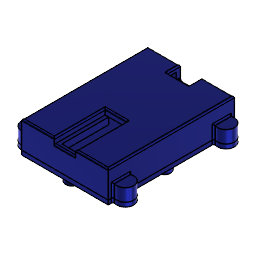
breadboard_case_CAD_v1 (Autodesk Fusion 360 design; units mm, degrees)
Autodesk Fusion 360 part; units mm, degrees
note: some values were not read from the file. Set by a fixed rule: which face or edge a step refers to.
(part 1 of 2)
sketch "breadboard_base" plane through (0, 0, 0) normal (0, 0, 1) x (1, 0, 0)
  line L0 (-27.2, 41.115) -> (27.2, 41.115)
  line L1 (27.2, 41.115) -> (27.2, -41.115)
  line L2 (27.2, -41.115) -> (-27.2, -41.115)
  line L3 (-27.2, -41.115) -> (-27.2, 41.115)
  dimension "d1" = 54.4
  dimension "d2" = 82.23
  dimension "d5" = 41.115
  dimension "d7" = 27.2
  constraint horizontal L0
  constraint vertical L1
  constraint horizontal L2
  constraint vertical L3
  measures "d1" distance of L0.start L0.end
  measures "d2" distance of L0.start L2.end
  measures "d5" distance of origin L0
  measures "d7" distance of origin L3
extrude "Extrude1" add sketch "breadboard_base" along normal blind 10 makes body 1
sketch "ravine_base" plane through (0, 0, 10) normal (0, 0, 1) x (-1, 0, 0)
  line L0 (27.2, 41.115) -> (-27.2, 41.115)
  line L1 (-27.2, 41.115) -> (-27.2, -41.115)
  line L2 (-27.2, -41.115) -> (27.2, -41.115)
  line L3 (27.2, -41.115) -> (27.2, 41.115)
  line L4 (1.5, -41.115) -> (-1.5, -41.115)
  line L5 (-1.5, -41.115) -> (-1.5, 41.115)
  line L6 (-1.5, 41.115) -> (1.5, 41.115)
  line L7 (1.5, 41.115) -> (1.5, -41.115)
  line L8 (0, -1.75) -> (0, -22.5)
  dimension "ravine_width" = 3
  constraint horizontal L4
  constraint vertical L5
  constraint horizontal L6
  constraint vertical L7
  constraint coincident L0 L5.end
  constraint coincident L2 L4.start
  constraint symmetric L5 L7 L8
  measures "ravine_width" distance of L5 L7
extrude "Extrude2" cut sketch "ravine_base" against normal blind 3 contours L0 L2 L4 L5 L6 L7 bodies 1
sketch "tab_base" plane through (0, 0, 0) normal (0, 0, 1) x (1, 0, 0)
  line L0 (-27.2, 41.115) -> (27.2, 41.115)
  line L1 (-27.2, -41.115) -> (-27.2, 41.115)
  line L2 (27.2, 41.115) -> (27.2, -41.115)
  line L3 (27.2, -41.115) -> (-27.2, -41.115)
  line L4 (1.5, 41.115) -> (1.5, -41.115)
  line L5 (1.5, -41.115) -> (27.2, -41.115)
  line L6 (1.5, -41.115) -> (-1.5, -41.115)
  line L7 (1.5, -41.115) -> (-1.5, -41.115)
  line L8 (-1.5, -41.115) -> (-1.5, -42.615)
  line L9 (-1.5, -42.615) -> (1.5, -42.615)
  line L10 (1.5, -42.615) -> (1.5, -41.115)
  line L11 (24.2, -41.115) -> (21.2, -41.115)
  line L12 (21.2, -41.115) -> (21.2, -42.615)
  line L13 (21.2, -42.615) -> (24.2, -42.615)
  line L14 (24.2, -42.615) -> (24.2, -41.115)
  line L15 (-21.2, -41.115) -> (-24.2, -41.115)
  line L16 (-24.2, -41.115) -> (-24.2, -42.615)
  line L17 (-24.2, -42.615) -> (-21.2, -42.615)
  line L18 (-21.2, -42.615) -> (-21.2, -41.115)
  line L19 (-27.2, -28.115) -> (-28.7, -28.115)
  line L20 (-28.7, -28.115) -> (-28.7, -25.115)
  line L21 (-28.7, -25.115) -> (-27.2, -25.115)
  line L22 (-27.2, -25.115) -> (-27.2, -28.115)
  line L23 (-27.2, 25.615) -> (-28.7, 25.615)
  line L24 (-28.7, 25.615) -> (-28.7, 28.615)
  line L25 (-28.7, 28.615) -> (-27.2, 28.615)
  line L26 (-27.2, 28.615) -> (-27.2, 25.615)
  dimension "d82" = 1.5
  dimension "d83" = 3
  dimension "d84" = 1.5
  dimension "d85" = 3
  dimension "d86" = 3
  dimension "d87" = 3
  dimension "d88" = 1.5
  dimension "d89" = 13
  dimension "d90" = 3
  dimension "d91" = 1.5
  dimension "d92" = 12.5
  dimension "d93" = 1.5
  dimension "d94" = 3
  constraint horizontal L7
  constraint vertical L8
  constraint horizontal L9
  constraint vertical L10
  constraint coincident L4.end L5.start
  constraint horizontal L11
  constraint vertical L12
  constraint horizontal L13
  constraint vertical L14
  constraint coincident L3 L11.start
  constraint horizontal L15
  constraint vertical L16
  constraint horizontal L17
  constraint vertical L18
  constraint coincident L3 L15.start
  constraint horizontal L19
  constraint vertical L20
  constraint horizontal L21
  constraint vertical L22
  constraint coincident L1 L19.start
  constraint horizontal L23
  constraint vertical L24
  constraint horizontal L25
  constraint vertical L26
  constraint coincident L1 L23.start
  measures "d82" distance of L6.end L8.end
  measures "d83" distance of L2.end L11.start
  measures "d84" distance of L11.end L12.end
  measures "d85" distance of L12.end L13.end
  measures "d86" distance of L1.start L15.end
  measures "d87" distance of L16.end L17.end
  measures "d88" distance of L15.start L17.end
  measures "d89" distance of L1.start L19
  measures "d90" distance of L19.end L20.end
  measures "d91" distance of L19.start L19.end
  measures "d92" distance of L0.start L25.end
  measures "d93" distance of L24.end L25.end
  measures "d94" distance of L23.end L24.end
extrude "Extrude3" add sketch "tab_base" along normal blind 5.1 contours L1 L23 L24 L25 L26 | L3 L6 L7 L8 L9 L10 | L3 L5 L11 L12 L13 L14 | L1 L19 L20 L21 L22 | L3 L15 L16 L17 L18 bodies 1
sketch "all_points" plane through (0, 0, 10) normal (0, 0, 1) x (-1, 0, 0)
  line L0 (1.5, 41.115) -> (1.5, -41.115)
  line L1 (1.5, -41.115) -> (27.2, -41.115)
  line L2 (27.2, -41.115) -> (27.2, 41.115)
  line L3 (27.2, 41.115) -> (1.5, 41.115)
  line L4 (0, 0) -> (27.2, 0) construction
  line L5 (-1.75, 0) -> (-22.5, 0)
  line L6 (0, -1.75) -> (0, -22.5)
  point P0 (3.8, -1.27)
  point P1 (6.34, -1.27)
  point P2 (8.88, -1.27)
  point P3 (11.42, -1.27)
  point P4 (13.96, -1.27)
  point P5 (3.8, -3.81)
  point P6 (6.34, -3.81)
  point P7 (8.88, -3.81)
  point P8 (11.42, -3.81)
  point P9 (13.96, -3.81)
  point P10 (3.8, -6.35)
  point P11 (6.34, -6.35)
  point P12 (8.88, -6.35)
  point P13 (11.42, -6.35)
  point P14 (13.96, -6.35)
  point P15 (3.8, -8.89)
  point P16 (6.34, -8.89)
  point P17 (8.88, -8.89)
  point P18 (11.42, -8.89)
  point P19 (13.96, -8.89)
  point P20 (3.8, -11.43)
  point P21 (6.34, -11.43)
  point P22 (8.88, -11.43)
  point P23 (11.42, -11.43)
  point P24 (13.96, -11.43)
  point P25 (3.8, -13.97)
  point P26 (6.34, -13.97)
  point P27 (8.88, -13.97)
  point P28 (11.42, -13.97)
  point P29 (13.96, -13.97)
  point P30 (3.8, -16.51)
  point P31 (6.34, -16.51)
  point P32 (8.88, -16.51)
  point P33 (11.42, -16.51)
  point P34 (13.96, -16.51)
  point P35 (3.8, -19.05)
  point P36 (6.34, -19.05)
  point P37 (8.88, -19.05)
  point P38 (11.42, -19.05)
  point P39 (13.96, -19.05)
  point P40 (3.8, -21.59)
  point P41 (6.34, -21.59)
  point P42 (8.88, -21.59)
  point P43 (11.42, -21.59)
  point P44 (13.96, -21.59)
  point P45 (3.8, -24.13)
  point P46 (6.34, -24.13)
  point P47 (8.88, -24.13)
  point P48 (11.42, -24.13)
  point P49 (13.96, -24.13)
  point P50 (3.8, -26.67)
  point P51 (6.34, -26.67)
  point P52 (8.88, -26.67)
  point P53 (11.42, -26.67)
  point P54 (13.96, -26.67)
  point P55 (3.8, -29.21)
  point P56 (6.34, -29.21)
  point P57 (8.88, -29.21)
  point P58 (11.42, -29.21)
  point P59 (13.96, -29.21)
  point P60 (3.8, -31.75)
  point P61 (6.34, -31.75)
  point P62 (8.88, -31.75)
  point P63 (11.42, -31.75)
  point P64 (13.96, -31.75)
  point P65 (3.8, -34.29)
  point P66 (6.34, -34.29)
  point P67 (8.88, -34.29)
  point P68 (11.42, -34.29)
  point P69 (13.96, -34.29)
  point P70 (3.8, -36.83)
  point P71 (6.34, -36.83)
  point P72 (8.88, -36.83)
  point P73 (11.42, -36.83)
  point P74 (13.96, -36.83)
  point P75 (20.71, 0)
  point P76 (20.71, -5.08)
  point P77 (23.25, -5.08)
  point P78 (20.71, -2.54)
  point P79 (23.25, -2.54)
  point P80 (23.25, 0)
  point P81 (20.71, 2.54)
  point P82 (23.25, 2.54)
  point P83 (20.71, 5.08)
  point P84 (23.25, 5.08)
  point P85 (23.25, -35.56)
  point P86 (23.25, -27.94)
  point P87 (20.71, -25.4)
  point P88 (23.25, -30.48)
  point P89 (20.71, -30.48)
  point P90 (23.25, -33.02)
  point P91 (20.71, -27.94)
  point P92 (20.71, -35.56)
  point P93 (23.25, -25.4)
  point P94 (20.71, -33.02)
  point P95 (23.25, -20.32)
  point P96 (23.25, -12.7)
  point P97 (20.71, -10.16)
  point P98 (23.25, -15.24)
  point P99 (20.71, -15.24)
  point P100 (23.25, -17.78)
  point P101 (20.71, -12.7)
  point P102 (20.71, -20.32)
  point P103 (23.25, -10.16)
  point P104 (20.71, -17.78)
  point P105 (23.25, 10.16)
  point P106 (23.25, 17.78)
  point P107 (20.71, 20.32)
  point P108 (23.25, 15.24)
  point P109 (20.71, 15.24)
  point P110 (23.25, 12.7)
  point P111 (20.71, 17.78)
  point P112 (20.71, 10.16)
  point P113 (23.25, 20.32)
  point P114 (20.71, 12.7)
  point P115 (23.25, 25.4)
  point P116 (23.25, 33.02)
  point P117 (20.71, 35.56)
  point P118 (23.25, 30.48)
  point P119 (20.71, 30.48)
  point P120 (23.25, 27.94)
  point P121 (20.71, 33.02)
  point P122 (20.71, 25.4)
  point P123 (23.25, 35.56)
  point P124 (20.71, 27.94)
  point P125 (6.34, 26.67)
  point P126 (13.96, 16.51)
  point P127 (3.8, 29.21)
  point P128 (13.96, 19.05)
  point P129 (6.34, 11.43)
  point P130 (8.88, 6.35)
  point P131 (3.8, 13.97)
  point P132 (6.34, 19.05)
  point P133 (3.8, 36.83)
  point P134 (8.88, 31.75)
  point P135 (13.96, 21.59)
  point P136 (3.8, 19.05)
  point P137 (6.34, 13.97)
  point P138 (3.8, 24.13)
  point P139 (13.96, 3.81)
  point P140 (6.34, 34.29)
  point P141 (13.96, 31.75)
  point P142 (6.34, 3.81)
  point P143 (13.96, 24.13)
  point P144 (11.42, 1.27)
  point P145 (13.96, 6.35)
  point P146 (8.88, 16.51)
  point P147 (11.42, 21.59)
  point P148 (6.34, 8.89)
  point P149 (6.34, 21.59)
  point P150 (6.34, 1.27)
  point P151 (8.88, 26.67)
  point P152 (11.42, 6.35)
  point P153 (13.96, 1.27)
  point P154 (3.8, 3.81)
  point P155 (3.8, 8.89)
  point P156 (8.88, 29.21)
  point P157 (6.34, 24.13)
  point P158 (13.96, 36.83)
  point P159 (11.42, 34.29)
  point P160 (8.88, 24.13)
  point P161 (3.8, 11.43)
  point P162 (11.42, 36.83)
  point P163 (11.42, 24.13)
  point P164 (11.42, 13.97)
  point P165 (13.96, 8.89)
  point P166 (6.34, 29.21)
  point P167 (6.34, 6.35)
  point P168 (8.88, 36.83)
  point P169 (11.42, 31.75)
  point P170 (3.8, 6.35)
  point P171 (8.88, 11.43)
  point P172 (6.34, 16.51)
  point P173 (3.8, 31.75)
  point P174 (13.96, 26.67)
  point P175 (8.88, 3.81)
  point P176 (8.88, 19.05)
  point P177 (8.88, 1.27)
  point P178 (13.96, 13.97)
  point P179 (8.88, 13.97)
  point P180 (6.34, 31.75)
  point P181 (8.88, 8.89)
  point P182 (11.42, 26.67)
  point P183 (3.8, 1.27)
  point P184 (11.42, 19.05)
  point P185 (13.96, 29.21)
  point P186 (11.42, 29.21)
  point P187 (3.8, 21.59)
  point P188 (13.96, 11.43)
  point P189 (11.42, 11.43)
  point P190 (13.96, 34.29)
  point P191 (3.8, 34.29)
  point P192 (11.42, 8.89)
  point P193 (11.42, 16.51)
  point P194 (11.42, 3.81)
  point P195 (3.8, 26.67)
  point P196 (8.88, 21.59)
  point P197 (8.88, 34.29)
  point P198 (6.34, 36.83)
  point P199 (3.8, 16.51)
  point P200 (-23.25, -15.24)
  point P201 (-3.8, 1.27)
  point P202 (-3.8, -29.21)
  point P203 (-23.25, -10.16)
  point P204 (-8.88, -24.13)
  point P205 (-8.88, 21.59)
  point P206 (-6.34, -13.97)
  point P207 (-20.71, 10.16)
  point P208 (-23.25, 15.24)
  point P209 (-6.34, 29.21)
  point P210 (-11.42, -24.13)
  point P211 (-23.25, -25.4)
  point P212 (-13.96, -11.43)
  point P213 (-3.8, -13.97)
  point P214 (-3.8, -8.89)
  point P215 (-3.8, -16.51)
  point P216 (-20.71, -35.56)
  point P217 (-13.96, -29.21)
  point P218 (-23.25, -30.48)
  point P219 (-3.8, -3.81)
  point P220 (-6.34, -19.05)
  point P221 (-20.71, -30.48)
  point P222 (-11.42, -36.83)
  point P223 (-6.34, -16.51)
  point P224 (-20.71, -27.94)
  point P225 (-6.34, 16.51)
  point P226 (-11.42, -31.75)
  point P227 (-20.71, 12.7)
  point P228 (-11.42, -6.35)
  point P229 (-13.96, -19.05)
  point P230 (-11.42, 31.75)
  point P231 (-20.71, 15.24)
  point P232 (-11.42, 8.89)
  point P233 (-13.96, -13.97)
  point P234 (-13.96, -16.51)
  point P235 (-8.88, -26.67)
  point P236 (-3.8, -34.29)
  point P237 (-3.8, 26.67)
  point P238 (-13.96, -26.67)
  point P239 (-13.96, 21.59)
  point P240 (-20.71, 17.78)
  point P241 (-3.8, 13.97)
  point P242 (-8.88, -31.75)
  point P243 (-6.34, -36.83)
  point P244 (-3.8, -19.05)
  point P245 (-20.71, -12.7)
  point P246 (-23.25, -35.56)
  point P247 (-11.42, -21.59)
  point P248 (-3.8, -26.67)
  point P249 (-13.96, -21.59)
  point P250 (-3.8, -6.35)
  point P251 (-20.71, -15.24)
  point P252 (-8.88, -21.59)
  point P253 (-6.34, -26.67)
  point P254 (-13.96, -36.83)
  point P255 (-11.42, -29.21)
  point P256 (-6.34, -34.29)
  point P257 (-3.8, 6.35)
  point P258 (-3.8, -1.27)
  point P259 (-20.71, -20.32)
  point P260 (-6.34, -21.59)
  point P261 (-8.88, -3.81)
  point P262 (-11.42, 29.21)
  point P263 (-13.96, -34.29)
  point P264 (-8.88, 8.89)
  point P265 (-23.25, 17.78)
  point P266 (-23.25, -12.7)
  point P267 (-3.8, -11.43)
  point P268 (-8.88, -16.51)
  point P269 (-3.8, 3.81)
  point P270 (-13.96, -31.75)
  point P271 (-11.42, -16.51)
  point P272 (-8.88, -19.05)
  point P273 (-8.88, -36.83)
  point P274 (-20.71, -25.4)
  point P275 (-23.25, -17.78)
  point P276 (-23.25, -27.94)
  point P277 (-6.34, -29.21)
  point P278 (-23.25, -33.02)
  point P279 (-23.25, -20.32)
  point P280 (-20.71, -33.02)
  point P281 (-23.25, 20.32)
  point P282 (-11.42, -11.43)
  point P283 (-6.34, 24.13)
  point P284 (-3.8, -21.59)
  point P285 (-3.8, 21.59)
  point P286 (-13.96, 34.29)
  point P287 (-6.34, 8.89)
  point P288 (-20.71, 20.32)
  point P289 (-11.42, -8.89)
  point P290 (-13.96, -24.13)
  point P291 (-8.88, -13.97)
  point P292 (-8.88, 29.21)
  point P293 (-6.34, -11.43)
  point P294 (-11.42, -13.97)
  point P295 (-23.25, 12.7)
  point P296 (-11.42, 19.05)
  point P297 (-11.42, 24.13)
  point P298 (-3.8, -36.83)
  point P299 (-20.71, 27.94)
  point P300 (-6.34, 21.59)
  point P301 (-20.71, 30.48)
  point P302 (-13.96, -1.27)
  point P303 (-11.42, 16.51)
  point P304 (-13.96, -6.35)
  point P305 (-13.96, 11.43)
  point P306 (-8.88, 16.51)
  point P307 (-11.42, 34.29)
  point P308 (-6.34, 36.83)
  point P309 (-23.25, 30.48)
  point P310 (-13.96, 24.13)
  point P311 (-6.34, 31.75)
  point P312 (-20.71, 35.56)
  point P313 (-3.8, -24.13)
  point P314 (-11.42, 3.81)
  point P315 (-6.34, 19.05)
  point P316 (-8.88, 11.43)
  point P317 (-3.8, 24.13)
  point P318 (-8.88, 34.29)
  point P319 (-23.25, -5.08)
  point P320 (-8.88, -34.29)
  point P321 (-8.88, 31.75)
  point P322 (-23.25, 33.02)
  point P323 (-6.34, -8.89)
  point P324 (-8.88, 19.05)
  point P325 (-8.88, 26.67)
  point P326 (-8.88, -29.21)
  point P327 (-6.34, 26.67)
  point P328 (-13.96, 26.67)
  point P329 (-6.34, -24.13)
  point P330 (-6.34, -31.75)
  point P331 (-11.42, -19.05)
  point P332 (-8.88, 36.83)
  point P333 (-11.42, 21.59)
  point P334 (-11.42, 6.35)
  point P335 (-20.71, 5.08)
  point P336 (-8.88, 24.13)
  point P337 (-11.42, -34.29)
  point P338 (-13.96, 8.89)
  point P339 (-3.8, 19.05)
  point P340 (-20.71, 0)
  point P341 (-3.8, 36.83)
  point P342 (-20.71, -17.78)
  point P343 (-13.96, 31.75)
  point P344 (-13.96, 13.97)
  point P345 (-23.25, 2.54)
  point P346 (-11.42, -26.67)
  point P347 (-20.71, -10.16)
  point P348 (-8.88, -11.43)
  point P349 (-3.8, 16.51)
  point P350 (-20.71, -5.08)
  point P351 (-23.25, 10.16)
  point P352 (-3.8, -31.75)
  point P353 (-13.96, 19.05)
  point P354 (-20.71, 25.4)
  point P355 (-20.71, 33.02)
  point P356 (-13.96, 36.83)
  point P357 (-11.42, 36.83)
  point P358 (-11.42, 26.67)
  point P359 (-6.34, 34.29)
  point P360 (-11.42, 11.43)
  point P361 (-6.34, 11.43)
  point P362 (-8.88, 13.97)
  point P363 (-3.8, 31.75)
  point P364 (-11.42, 13.97)
  point P365 (-23.25, 5.08)
  point P366 (-23.25, 27.94)
  point P367 (-13.96, 29.21)
  point P368 (-3.8, 8.89)
  point P369 (-3.8, 29.21)
  point P370 (-23.25, 25.4)
  point P371 (-3.8, 11.43)
  point P372 (-3.8, 34.29)
  point P373 (-6.34, 13.97)
  point P374 (-13.96, 6.35)
  point P375 (-8.88, 3.81)
  point P376 (-8.88, -6.35)
  point P377 (-13.96, 16.51)
  point P378 (-11.42, 1.27)
  point P379 (-23.25, 35.56)
  point P380 (-13.96, 1.27)
  point P381 (-8.88, 1.27)
  point P382 (-13.96, -3.81)
  point P383 (-6.34, -3.81)
  point P384 (-23.25, 0)
  point P385 (-8.88, -1.27)
  point P386 (-6.34, -6.35)
  point P387 (-23.25, -2.54)
  point P388 (-6.34, 3.81)
  point P389 (-6.34, 1.27)
  point P390 (-6.34, -1.27)
  point P391 (-20.71, 2.54)
  point P392 (-13.96, 3.81)
  point P393 (-13.96, -8.89)
  point P394 (-11.42, -3.81)
  point P395 (-20.71, -2.54)
  point P396 (-11.42, -1.27)
  point P397 (-8.88, 6.35)
  point P398 (-6.34, 6.35)
  point P399 (-8.88, -8.89)
  dimension "d30" = 1.27
  dimension "d31" = 3.8
  dimension "d35" = 10.16
  dimension "d36" = -35.56
  dimension "d37" = 6.75
  dimension "d40" = 2.54
  dimension "d41" = 5.08
  dimension "d44" = 0
  dimension "d45" = 30.48
  constraint coincident L4.start origin
  constraint midpoint L2 L4.end
  constraint coincident L4 P75
  constraint symmetric P0 L5 P183
  constraint symmetric P1 L5 P150
  constraint symmetric P2 L5 P177
  constraint symmetric P3 L5 P144
  constraint symmetric P4 L5 P153
  constraint symmetric P5 L5 P154
  constraint symmetric P6 L5 P142
  constraint symmetric P7 L5 P175
  constraint symmetric P8 L5 P194
  constraint symmetric P9 L5 P139
  constraint symmetric P10 L5 P170
  constraint symmetric P11 L5 P167
  constraint symmetric P12 L5 P130
  constraint symmetric P13 L5 P152
  constraint symmetric P14 L5 P145
  constraint symmetric P15 L5 P155
  constraint symmetric P16 L5 P148
  constraint symmetric P17 L5 P181
  constraint symmetric P18 L5 P192
  constraint symmetric P19 L5 P165
  constraint symmetric P20 L5 P161
  constraint symmetric P21 L5 P129
  constraint symmetric P22 L5 P171
  constraint symmetric P23 L5 P189
  constraint symmetric P24 L5 P188
  constraint symmetric P25 L5 P131
  constraint symmetric P26 L5 P137
  constraint symmetric P27 L5 P179
  constraint symmetric P28 L5 P164
  constraint symmetric P29 L5 P178
  constraint symmetric P30 L5 P199
  constraint symmetric P31 L5 P172
  constraint symmetric P32 L5 P146
  constraint symmetric P33 L5 P193
  constraint symmetric P34 L5 P126
  constraint symmetric P35 L5 P136
  constraint symmetric P36 L5 P132
  constraint symmetric P37 L5 P176
  constraint symmetric P38 L5 P184
  constraint symmetric P39 L5 P128
  constraint symmetric P40 L5 P187
  constraint symmetric P41 L5 P149
  constraint symmetric P42 L5 P196
  constraint symmetric P43 L5 P147
  constraint symmetric P44 L5 P135
  constraint symmetric P45 L5 P138
  constraint symmetric P46 L5 P157
  constraint symmetric P47 L5 P160
  constraint symmetric P48 L5 P163
  constraint symmetric P49 L5 P143
  constraint symmetric P50 L5 P195
  constraint symmetric P51 L5 P125
  constraint symmetric P52 L5 P151
  constraint symmetric P53 L5 P182
  constraint symmetric P54 L5 P174
  constraint symmetric P55 L5 P127
  constraint symmetric P56 L5 P166
  constraint symmetric P57 L5 P156
  constraint symmetric P58 L5 P186
  constraint symmetric P59 L5 P185
  constraint symmetric P60 L5 P173
  constraint symmetric P61 L5 P180
  constraint symmetric P62 L5 P134
  constraint symmetric P63 L5 P169
  constraint symmetric P64 L5 P141
  constraint symmetric P65 L5 P191
  constraint symmetric P66 L5 P140
  constraint symmetric P67 L5 P197
  constraint symmetric P68 L5 P159
  constraint symmetric P69 L5 P190
  constraint symmetric P70 L5 P133
  constraint symmetric P71 L5 P198
  constraint symmetric P72 L5 P168
  constraint symmetric P73 L5 P162
  constraint symmetric P74 L5 P158
  constraint symmetric P0 L6 P258
  constraint symmetric P1 L6 P390
  constraint symmetric P2 L6 P385
  constraint symmetric P3 L6 P396
  constraint symmetric P4 L6 P302
  constraint symmetric P5 L6 P219
  constraint symmetric P6 L6 P383
  constraint symmetric P7 L6 P261
  constraint symmetric P8 L6 P394
  constraint symmetric P9 L6 P382
  constraint symmetric P10 L6 P250
  constraint symmetric P11 L6 P386
  constraint symmetric P12 L6 P376
  constraint symmetric P13 L6 P228
  constraint symmetric P14 L6 P304
  constraint symmetric P15 L6 P214
  constraint symmetric P16 L6 P323
  constraint symmetric P17 L6 P399
  constraint symmetric P18 L6 P289
  constraint symmetric P19 L6 P393
  constraint symmetric P20 L6 P267
  constraint symmetric P21 L6 P293
  constraint symmetric P22 L6 P348
  constraint symmetric P23 L6 P282
  constraint symmetric P24 L6 P212
  constraint symmetric P25 L6 P213
  constraint symmetric P26 L6 P206
  constraint symmetric P27 L6 P291
  constraint symmetric P28 L6 P294
  constraint symmetric P29 L6 P233
  constraint symmetric P30 L6 P215
  constraint symmetric P31 L6 P223
  constraint symmetric P32 L6 P268
  constraint symmetric P33 L6 P271
  constraint symmetric P34 L6 P234
  constraint symmetric P35 L6 P244
  constraint symmetric P36 L6 P220
  constraint symmetric P37 L6 P272
  constraint symmetric P38 L6 P331
  constraint symmetric P39 L6 P229
  constraint symmetric P40 L6 P284
  constraint symmetric P41 L6 P260
  constraint symmetric P42 L6 P252
  constraint symmetric P43 L6 P247
  constraint symmetric P44 L6 P249
  constraint symmetric P45 L6 P313
  constraint symmetric P46 L6 P329
  constraint symmetric P47 L6 P204
  constraint symmetric P48 L6 P210
  constraint symmetric P49 L6 P290
  constraint symmetric P50 L6 P248
  constraint symmetric P51 L6 P253
  constraint symmetric P52 L6 P235
  constraint symmetric P53 L6 P346
  constraint symmetric P54 L6 P238
  constraint symmetric P55 L6 P202
  constraint symmetric P56 L6 P277
  constraint symmetric P57 L6 P326
  constraint symmetric P58 L6 P255
  constraint symmetric P59 L6 P217
  constraint symmetric P60 L6 P352
  constraint symmetric P61 L6 P330
  constraint symmetric P62 L6 P242
  constraint symmetric P63 L6 P226
  constraint symmetric P64 L6 P270
  constraint symmetric P65 L6 P236
  constraint symmetric P66 L6 P256
  constraint symmetric P67 L6 P320
  constraint symmetric P68 L6 P337
  constraint symmetric P69 L6 P263
  constraint symmetric P70 L6 P298
  constraint symmetric P71 L6 P243
  constraint symmetric P72 L6 P273
  constraint symmetric P73 L6 P222
  constraint symmetric P74 L6 P254
  constraint symmetric P75 L6 P340
  constraint symmetric P76 L6 P350
  constraint symmetric P77 L6 P319
  constraint symmetric P78 L6 P395
  constraint symmetric P79 L6 P387
  constraint symmetric P80 L6 P384
  constraint symmetric P81 L6 P391
  constraint symmetric P82 L6 P345
  constraint symmetric P83 L6 P335
  constraint symmetric P84 L6 P365
  constraint symmetric P85 L6 P246
  constraint symmetric P86 L6 P276
  constraint symmetric P87 L6 P274
  constraint symmetric P88 L6 P218
  constraint symmetric P89 L6 P221
  constraint symmetric P90 L6 P278
  constraint symmetric P91 L6 P224
  constraint symmetric P92 L6 P216
  constraint symmetric P93 L6 P211
  constraint symmetric P94 L6 P280
  constraint symmetric P95 L6 P279
  constraint symmetric P96 L6 P266
  constraint symmetric P97 L6 P347
  constraint symmetric P98 L6 P200
  constraint symmetric P99 L6 P251
  constraint symmetric P100 L6 P275
  constraint symmetric P101 L6 P245
  constraint symmetric P102 L6 P259
  constraint symmetric P103 L6 P203
  constraint symmetric P104 L6 P342
  constraint symmetric P105 L6 P351
  constraint symmetric P106 L6 P265
  constraint symmetric P107 L6 P288
  constraint symmetric P108 L6 P208
  constraint symmetric P109 L6 P231
  constraint symmetric P110 L6 P295
  constraint symmetric P111 L6 P240
  constraint symmetric P112 L6 P207
  constraint symmetric P113 L6 P281
  constraint symmetric P114 L6 P227
  constraint symmetric P115 L6 P370
  constraint symmetric P116 L6 P322
  constraint symmetric P117 L6 P312
  constraint symmetric P118 L6 P309
  constraint symmetric P119 L6 P301
  constraint symmetric P120 L6 P366
  constraint symmetric P121 L6 P355
  constraint symmetric P122 L6 P354
  constraint symmetric P123 L6 P379
  constraint symmetric P124 L6 P299
  constraint symmetric P125 L6 P327
  constraint symmetric P126 L6 P377
  constraint symmetric P127 L6 P369
  constraint symmetric P128 L6 P353
  constraint symmetric P129 L6 P361
  constraint symmetric P130 L6 P397
  constraint symmetric P131 L6 P241
  constraint symmetric P132 L6 P315
  constraint symmetric P133 L6 P341
  constraint symmetric P134 L6 P321
  constraint symmetric P135 L6 P239
  constraint symmetric P136 L6 P339
  constraint symmetric P137 L6 P373
  constraint symmetric P138 L6 P317
  constraint symmetric P139 L6 P392
  constraint symmetric P140 L6 P359
  constraint symmetric P141 L6 P343
  constraint symmetric P142 L6 P388
  constraint symmetric P143 L6 P310
  constraint symmetric P144 L6 P378
  constraint symmetric P145 L6 P374
  constraint symmetric P146 L6 P306
  constraint symmetric P147 L6 P333
  constraint symmetric P148 L6 P287
  constraint symmetric P149 L6 P300
  constraint symmetric P150 L6 P389
  constraint symmetric P151 L6 P325
  constraint symmetric P152 L6 P334
  constraint symmetric P153 L6 P380
  constraint symmetric P154 L6 P269
  constraint symmetric P155 L6 P368
  constraint symmetric P156 L6 P292
  constraint symmetric P157 L6 P283
  constraint symmetric P158 L6 P356
  constraint symmetric P159 L6 P307
  constraint symmetric P160 L6 P336
  constraint symmetric P161 L6 P371
  constraint symmetric P162 L6 P357
  constraint symmetric P163 L6 P297
  constraint symmetric P164 L6 P364
  constraint symmetric P165 L6 P338
  constraint symmetric P166 L6 P209
  constraint symmetric P167 L6 P398
  constraint symmetric P168 L6 P332
  constraint symmetric P169 L6 P230
  constraint symmetric P170 L6 P257
  constraint symmetric P171 L6 P316
  constraint symmetric P172 L6 P225
  constraint symmetric P173 L6 P363
  constraint symmetric P174 L6 P328
  constraint symmetric P175 L6 P375
  constraint symmetric P176 L6 P324
  constraint symmetric P177 L6 P381
  constraint symmetric P178 L6 P344
  constraint symmetric P179 L6 P362
  constraint symmetric P180 L6 P311
  constraint symmetric P181 L6 P264
  constraint symmetric P182 L6 P358
  constraint symmetric P183 L6 P201
  constraint symmetric P184 L6 P296
  constraint symmetric P185 L6 P367
  constraint symmetric P186 L6 P262
  constraint symmetric P187 L6 P285
  constraint symmetric P188 L6 P305
  constraint symmetric P189 L6 P360
  constraint symmetric P190 L6 P286
  constraint symmetric P191 L6 P372
  constraint symmetric P192 L6 P232
  constraint symmetric P193 L6 P303
  constraint symmetric P194 L6 P314
  constraint symmetric P195 L6 P237
  constraint symmetric P196 L6 P205
  constraint symmetric P197 L6 P318
  constraint symmetric P198 L6 P308
  constraint symmetric P199 L6 P349
  measures "d30" vertical distance of L4.start P0
  measures "d31" horizontal distance of L4.start P0
  measures "d37" horizontal distance of P4 P75
hole "Hole1" at (-23.25, 20.32, 10) at (-23.25, 33.02, 10) at (-3.8, 8.89, 10) at (-23.25, -20.32, 10) at (-11.42, -19.05, 10) at (-8.88, 3.81, 10) at (-11.42, -26.67, 10) at (-11.42, -13.97, 10) at (-20.71, -5.08, 10) at (-8.88, -29.21, 10) at (-3.8, -19.05, 10) at (-13.96, -24.13, 10) at (-13.96, 26.67, 10) at (-3.8, -34.29, 10) at (-11.42, 6.35, 10) at (-3.8, -36.83, 10) at (-8.88, 34.29, 10) at (-23.25, 10.16, 10) at (-3.8, -13.97, 10) at (-6.34, 13.97, 10) at (-6.34, 29.21, 10) at (-11.42, -16.51, 10) at (-23.25, 5.08, 10) at (-23.25, -15.24, 10) at (-20.71, -17.78, 10) at (-3.8, 16.51, 10) at (-23.25, -10.16, 10) at (-6.34, 11.43, 10) at (-11.42, 21.59, 10) at (-20.71, 2.54, 10) at (-20.71, 17.78, 10) at (-13.96, 3.81, 10) at (-11.42, 36.83, 10) at (-6.34, 3.81, 10) at (-6.34, -19.05, 10) at (-3.8, 6.35, 10) at (-3.8, 36.83, 10) at (-20.71, 20.32, 10) at (-20.71, 25.4, 10) at (-11.42, -21.59, 10) at (-3.8, -6.35, 10) at (-3.8, 3.81, 10) at (-20.71, 33.02, 10) at (-23.25, 27.94, 10) at (-13.96, 21.59, 10) at (-23.25, 30.48, 10) at (-3.8, -1.27, 10) at (-8.88, -6.35, 10) at (-6.34, -13.97, 10) at (-11.42, 3.81, 10) at (-11.42, -34.29, 10) at (-6.34, 19.05, 10) at (-3.8, -11.43, 10) at (-11.42, 8.89, 10) at (-13.96, 34.29, 10) at (-6.34, 1.27, 10) at (-8.88, -1.27, 10) at (-13.96, -26.67, 10) at (-23.25, 17.78, 10) at (-6.34, 16.51, 10) at (-23.25, -25.4, 10) at (-13.96, -31.75, 10) at (-13.96, -29.21, 10) at (-23.25, -27.94, 10) at (-8.88, -16.51, 10) at (-8.88, -13.97, 10) at (-8.88, 31.75, 10) at (-8.88, 1.27, 10) at (-13.96, 16.51, 10) at (-11.42, 31.75, 10) at (-13.96, 11.43, 10) at (-20.71, -35.56, 10) at (-8.88, -11.43, 10) at (-13.96, 29.21, 10) at (-8.88, 24.13, 10) at (-8.88, 11.43, 10) at (-3.8, -8.89, 10) at (-8.88, 36.83, 10) at (-6.34, -3.81, 10) at (-8.88, -8.89, 10) at (-20.71, 10.16, 10) at (-13.96, -13.97, 10) at (-8.88, 19.05, 10) at (-6.34, -31.75, 10) at (-3.8, 19.05, 10) at (-6.34, 8.89, 10) at (-13.96, 24.13, 10) at (-6.34, -34.29, 10) at (-8.88, 26.67, 10) at (-11.42, 1.27, 10) at (-11.42, 24.13, 10) at (-6.34, -6.35, 10) at (-13.96, -19.05, 10) at (-3.8, -29.21, 10) at (-8.88, -34.29, 10) at (-3.8, 29.21, 10) at (-6.34, 26.67, 10) at (-6.34, -8.89, 10) at (-8.88, -31.75, 10) at (-11.42, 11.43, 10) at (-13.96, -1.27, 10) at (-8.88, -36.83, 10) at (-8.88, 21.59, 10) at (-23.25, 35.56, 10) at (-13.96, -8.89, 10) at (-11.42, 34.29, 10) at (-20.71, -25.4, 10) at (-13.96, 1.27, 10) at (-23.25, 25.4, 10) at (-8.88, -3.81, 10) at (-8.88, 8.89, 10) at (-13.96, -11.43, 10) at (-3.8, -16.51, 10) at (-3.8, 21.59, 10) at (-11.42, -11.43, 10) at (-6.34, 31.75, 10) at (-20.71, -2.54, 10) at (-6.34, -36.83, 10) at (-20.71, -10.16, 10) at (-20.71, 5.08, 10) at (-23.25, 12.7, 10) at (-11.42, 19.05, 10) at (-3.8, 11.43, 10) at (-20.71, -15.24, 10) at (-8.88, -24.13, 10) at (-13.96, -16.51, 10) at (-8.88, -26.67, 10) at (-11.42, 16.51, 10) at (-8.88, 13.97, 10) at (-6.34, 6.35, 10) at (-23.25, -17.78, 10) at (-3.8, 13.97, 10) at (-3.8, 34.29, 10) at (-23.25, 0, 10) at (-11.42, -36.83, 10) at (-13.96, 8.89, 10) at (-20.71, 15.24, 10) at (-13.96, 36.83, 10) at (-23.25, -5.08, 10) at (-13.96, -36.83, 10) at (-11.42, 26.67, 10) at (-6.34, -26.67, 10) at (-20.71, -12.7, 10) at (-23.25, -12.7, 10) at (-13.96, 6.35, 10) at (-3.8, -24.13, 10) at (-20.71, -27.94, 10) at (-6.34, 36.83, 10) at (-8.88, 6.35, 10) at (-8.88, -21.59, 10) at (-11.42, -24.13, 10) at (-20.71, -30.48, 10) at (-8.88, 29.21, 10) at (-20.71, -33.02, 10) at (-6.34, -24.13, 10) at (-3.8, 24.13, 10) at (-6.34, -21.59, 10) at (-11.42, -3.81, 10) at (-13.96, -21.59, 10) at (-11.42, -1.27, 10) at (-3.8, -26.67, 10) at (-11.42, 29.21, 10) at (-23.25, -35.56, 10) at (-11.42, -29.21, 10) at (-20.71, 0, 10) at (-8.88, -19.05, 10) at (-23.25, -33.02, 10) at (-13.96, 31.75, 10) at (-6.34, 21.59, 10) at (-23.25, -30.48, 10) at (-6.34, -29.21, 10) at (-3.8, -21.59, 10) at (-11.42, -6.35, 10) at (-3.8, -3.81, 10) at (-20.71, 35.56, 10) at (-20.71, 30.48, 10) at (-11.42, -8.89, 10) at (-6.34, 24.13, 10) at (-3.8, 1.27, 10) at (-3.8, 26.67, 10) at (-6.34, -11.43, 10) at (-6.34, 34.29, 10) at (-6.34, -1.27, 10) at (-23.25, 2.54, 10) at (-20.71, 27.94, 10) at (-3.8, 31.75, 10) at (-6.34, -16.51, 10) at (-8.88, 16.51, 10) at (-13.96, 19.05, 10) at (-11.42, 13.97, 10) at (-13.96, -34.29, 10) at (-13.96, -6.35, 10) at (-23.25, 15.24, 10) at (-20.71, -20.32, 10) at (-3.8, -31.75, 10) at (-23.25, -2.54, 10) at (-13.96, 13.97, 10) at (-20.71, 12.7, 10) at (-13.96, -3.81, 10) at (-11.42, -31.75, 10) at (8.88, 16.51, 10) at (23.25, 35.56, 10) at (13.96, 24.13, 10) at (11.42, 31.75, 10) at (8.88, 3.81, 10) at (6.34, 16.51, 10) at (20.71, 15.24, 10) at (13.96, 8.89, 10) at (23.25, 12.7, 10) at (13.96, 1.27, 10) at (6.34, 36.83, 10) at (3.8, 19.05, 10) at (8.88, 13.97, 10) at (3.8, 24.13, 10) at (3.8, 11.43, 10) at (8.88, 29.21, 10) at (3.8, 29.21, 10) at (13.96, 16.51, 10) at (20.71, 17.78, 10) at (11.42, 21.59, 10) at (13.96, 26.67, 10) at (13.96, 36.83, 10) at (11.42, 24.13, 10) at (13.96, 19.05, 10) at (3.8, 21.59, 10) at (8.88, 34.29, 10) at (11.42, 36.83, 10) at (11.42, 19.05, 10) at (13.96, 21.59, 10) at (13.96, 34.29, 10) at (11.42, 6.35, 10) at (13.96, 3.81, 10) at (3.8, 3.81, 10) at (8.88, 1.27, 10) at (6.34, 24.13, 10) at (20.71, 33.02, 10) at (3.8, 8.89, 10) at (3.8, 36.83, 10) at (11.42, 3.81, 10) at (11.42, 34.29, 10) at (6.34, 11.43, 10) at (8.88, 24.13, 10) at (11.42, 16.51, 10) at (13.96, 29.21, 10) at (13.96, 6.35, 10) at (11.42, 26.67, 10) at (6.34, 19.05, 10) at (11.42, 13.97, 10) at (8.88, 26.67, 10) at (3.8, 1.27, 10) at (13.96, 11.43, 10) at (8.88, 31.75, 10) at (20.71, 10.16, 10) at (3.8, 13.97, 10) at (13.96, 31.75, 10) at (6.34, 21.59, 10) at (3.8, 26.67, 10) at (6.34, 29.21, 10) at (11.42, 29.21, 10) at (8.88, 21.59, 10) at (3.8, 31.75, 10) at (20.71, 5.08, 10) at (8.88, 36.83, 10) at (3.8, 6.35, 10) at (23.25, 5.08, 10) at (13.96, 13.97, 10) at (6.34, 3.81, 10) at (20.71, 25.4, 10) at (6.34, 31.75, 10) at (23.25, 20.32, 10) at (6.34, 1.27, 10) at (11.42, 1.27, 10) at (6.34, 34.29, 10) at (20.71, 35.56, 10) at (23.25, 2.54, 10) at (8.88, 6.35, 10) at (8.88, 8.89, 10) at (6.34, 6.35, 10) at (20.71, 2.54, 10) at (6.34, 13.97, 10) at (23.25, 17.78, 10) at (6.34, 26.67, 10) at (8.88, 11.43, 10) at (23.25, 33.02, 10) at (23.25, 10.16, 10) at (3.8, 16.51, 10) at (23.25, 27.94, 10) at (11.42, 8.89, 10) at (20.71, 27.94, 10) at (20.71, 20.32, 10) at (6.34, 8.89, 10) at (20.71, 30.48, 10) at (8.88, 19.05, 10) at (23.25, 30.48, 10) at (23.25, 25.4, 10) at (23.25, 15.24, 10) at (3.8, 34.29, 10) at (11.42, 11.43, 10) at (20.71, 12.7, 10) at (6.34, -34.29, 10) at (8.88, -19.05, 10) at (11.42, -29.21, 10) at (13.96, -1.27, 10) at (6.34, -21.59, 10) at (13.96, -19.05, 10) at (6.34, -19.05, 10) at (8.88, -8.89, 10) at (13.96, -16.51, 10) at (8.88, -13.97, 10) at (8.88, -11.43, 10) at (8.88, -16.51, 10) at (11.42, -24.13, 10) at (3.8, -16.51, 10) at (11.42, -6.35, 10) at (13.96, -6.35, 10) at (3.8, -19.05, 10) at (8.88, -31.75, 10) at (20.71, -35.56, 10) at (23.25, -5.08, 10) at (20.71, -12.7, 10) at (13.96, -13.97, 10) at (11.42, -1.27, 10) at (23.25, -10.16, 10) at (11.42, -11.43, 10) at (20.71, -10.16, 10) at (6.34, -36.83, 10) at (23.25, -20.32, 10) at (23.25, -33.02, 10) at (13.96, -3.81, 10) at (23.25, -35.56, 10) at (20.71, -30.48, 10) at (6.34, -1.27, 10) at (20.71, -25.4, 10) at (11.42, -16.51, 10) at (3.8, -8.89, 10) at (11.42, -19.05, 10) at (3.8, -6.35, 10) at (8.88, -3.81, 10) at (23.25, -12.7, 10) at (8.88, -1.27, 10) at (6.34, -8.89, 10) at (13.96, -8.89, 10) at (3.8, -1.27, 10) at (20.71, -20.32, 10) at (11.42, -3.81, 10) at (6.34, -3.81, 10) at (13.96, -26.67, 10) at (23.25, -15.24, 10) at (3.8, -29.21, 10) at (20.71, -5.08, 10) at (23.25, -2.54, 10) at (6.34, -6.35, 10) at (20.71, -33.02, 10) at (20.71, -15.24, 10) at (3.8, -3.81, 10) at (20.71, -2.54, 10) at (23.25, -27.94, 10) at (23.25, -17.78, 10) at (3.8, -11.43, 10) at (6.34, -29.21, 10) at (20.71, -27.94, 10) at (20.71, -17.78, 10) at (8.88, -6.35, 10) at (23.25, -25.4, 10) at (3.8, -36.83, 10) at (23.25, -30.48, 10) at (11.42, -13.97, 10) at (13.96, -36.83, 10) at (13.96, -11.43, 10) at (11.42, -31.75, 10) at (6.34, -31.75, 10) at (13.96, -31.75, 10) at (13.96, -34.29, 10) at (6.34, -13.97, 10) at (6.34, -11.43, 10) at (3.8, -26.67, 10) at (8.88, -24.13, 10) at (11.42, -36.83, 10) at (11.42, -34.29, 10) at (13.96, -29.21, 10) at (3.8, -21.59, 10) at (8.88, -21.59, 10) at (11.42, -8.89, 10) at (3.8, -31.75, 10) at (8.88, -34.29, 10) at (3.8, -24.13, 10) at (8.88, -26.67, 10) at (11.42, -26.67, 10) at (6.34, -16.51, 10) at (13.96, -24.13, 10) at (11.42, -21.59, 10) at (8.88, -36.83, 10) at (13.96, -21.59, 10) at (3.8, -13.97, 10) at (6.34, -24.13, 10) at (3.8, -34.29, 10) at (6.34, -26.67, 10) at (8.88, -29.21, 10) at (20.71, 0, 10) at (23.25, 0, 10) direction (0, 0, -1) diameter 1.524 depth 7 tip angle 180 bodies 1
chamfer "Chamfer2" distance 0.4 angle 45 8 edges at (-14.35, -41.115, 10) (-1.5, 0, 10) (-27.2, 0, 10) (-14.35, 41.115, 10) (14.35, 41.115, 10) (1.5, 0, 10) (27.2, 0, 10) (14.35, -41.115, 10) on bodies 1
sketch "case_wall" plane through (0, 0, 0) normal (0, 0, -1) x (1, 0, 0)
  line L0 (27.2, 41.115) -> (24.2, 41.115)
  line L1 (-27.2, 41.115) -> (-27.2, 28.115)
  line L2 (-27.2, -41.115) -> (27.2, -41.115)
  line L3 (27.2, -41.115) -> (27.2, 41.115)
  line L4 (-30.45, 44.365) -> (30.5, 44.365)
  line L5 (30.5, 44.365) -> (30.5, -44.415)
  line L6 (30.5, -44.415) -> (-30.45, -44.415)
  line L7 (-30.45, -44.415) -> (-30.45, 44.365)
  line L8 (24.2, 41.115) -> (24.2, 42.615)
  line L9 (24.2, 42.615) -> (21.2, 42.615)
  line L10 (21.2, 42.615) -> (21.2, 41.115)
  line L11 (-21.2, 41.115) -> (-21.2, 42.615)
  line L12 (-21.2, 42.615) -> (-24.2, 42.615)
  line L13 (-24.2, 42.615) -> (-24.2, 41.115)
  line L14 (21.2, 41.115) -> (1.5, 41.115)
  line L15 (1.5, 41.115) -> (1.5, 42.615)
  line L16 (1.5, 42.615) -> (-1.5, 42.615)
  line L17 (-1.5, 42.615) -> (-1.5, 41.115)
  line L18 (-1.5, 41.115) -> (-21.2, 41.115)
  line L19 (-24.2, 41.115) -> (-27.2, 41.115)
  line L20 (-27.2, 28.115) -> (-28.7, 28.115)
  line L21 (-28.7, 28.115) -> (-28.7, 25.115)
  line L22 (-28.7, 25.115) -> (-27.2, 25.115)
  line L23 (-27.2, 25.115) -> (-27.2, -25.615)
  line L24 (-27.2, -25.615) -> (-28.7, -25.615)
  line L25 (-28.7, -25.615) -> (-28.7, -28.615)
  line L26 (-28.7, -28.615) -> (-27.2, -28.615)
  line L27 (-27.2, -28.615) -> (-27.2, -41.115)
  line L28 (-27.5, -41.415) -> (27.5, -41.415)
  line L29 (27.5, -41.415) -> (27.5, 41.415)
  line L30 (27.5, 41.415) -> (24.5, 41.415)
  line L31 (24.5, 41.415) -> (24.5, 42.915)
  line L32 (24.5, 42.915) -> (20.9, 42.915)
  line L33 (20.9, 42.915) -> (20.9, 41.415)
  line L34 (20.9, 41.415) -> (1.8, 41.415)
  line L35 (1.8, 41.415) -> (1.8, 42.915)
  line L36 (1.8, 42.915) -> (-1.8, 42.915)
  line L37 (-1.8, 42.915) -> (-1.8, 41.415)
  line L38 (-1.8, 41.415) -> (-20.9, 41.415)
  line L39 (-20.9, 41.415) -> (-20.9, 42.915)
  line L40 (-20.9, 42.915) -> (-24.5, 42.915)
  line L41 (-24.5, 42.915) -> (-24.5, 41.415)
  line L42 (-24.5, 41.415) -> (-27.5, 41.415)
  line L43 (-27.5, 41.415) -> (-27.5, 28.415)
  line L44 (-27.5, 28.415) -> (-29, 28.415)
  line L45 (-29, 28.415) -> (-29, 24.815)
  line L46 (-29, 24.815) -> (-27.5, 24.815)
  line L47 (-27.5, 24.815) -> (-27.5, -25.315)
  line L48 (-27.5, -25.315) -> (-29, -25.315)
  line L49 (-29, -25.315) -> (-29, -28.915)
  line L50 (-29, -28.915) -> (-27.5, -28.915)
  line L51 (-27.5, -28.915) -> (-27.5, -41.415)
  dimension "d59" = 0.3
  dimension "d61" = 3
  dimension "d62" = 3
  constraint horizontal L4
  constraint vertical L5
  constraint horizontal L6
  constraint vertical L7
  measures "d61" distance of L6 L28
  measures "d62" distance of L5 L29
extrude "Extrude4" add sketch "case_wall" against normal blind 16 separate body contours L4 L5 L6 L7 makes body 2
ref_plane "WorkPlane1" through (-27.95, -26.615, 5.4) normal (0, 0, 1) x (1, 0, 0)
sketch "tab_top" plane through (0, 0, 5.4) normal (0, 0, 1) x (1, 0, 0)
  line L0 (-27.5, 28.915) -> (-27.5, 41.415)
  line L1 (-27.5, 41.415) -> (27.5, 41.415)
  line L2 (27.5, 41.415) -> (27.5, -41.415)
  line L3 (27.5, -41.415) -> (24.5, -41.415)
  line L4 (24.5, -41.415) -> (24.5, -42.915)
  line L5 (24.5, -42.915) -> (20.9, -42.915)
  line L6 (20.9, -42.915) -> (20.9, -41.415)
  line L7 (20.9, -41.415) -> (1.8, -41.415)
  line L8 (1.8, -41.415) -> (1.8, -42.915)
  line L9 (1.8, -42.915) -> (-1.8, -42.915)
  line L10 (-1.8, -42.915) -> (-1.8, -41.415)
  line L11 (-1.8, -41.415) -> (-20.9, -41.415)
  line L12 (-20.9, -41.415) -> (-20.9, -42.915)
  line L13 (-20.9, -42.915) -> (-24.5, -42.915)
  line L14 (-24.5, -42.915) -> (-24.5, -41.415)
  line L15 (-24.5, -41.415) -> (-27.5, -41.415)
  line L16 (-27.5, -41.415) -> (-27.5, -28.415)
  line L17 (-27.5, -28.415) -> (-29, -28.415)
  line L18 (-29, -28.415) -> (-29, -24.815)
  line L19 (-29, -24.815) -> (-27.5, -24.815)
  line L20 (-27.5, -24.815) -> (-27.5, 25.315)
  line L21 (-27.5, 25.315) -> (-29, 25.315)
  line L22 (-29, 25.315) -> (-29, 28.915)
  line L23 (-29, 28.915) -> (-27.5, 28.915)
  line L24 (30.5, 44.415) -> (-30.45, 44.415)
  line L25 (-30.45, 44.415) -> (-30.45, -44.365)
  line L26 (-30.45, -44.365) -> (30.5, -44.365)
  line L27 (30.5, -44.365) -> (30.5, 44.415)
  line L28 (-27.5, 25.1988) -> (-27.5, 28.915)
  line L29 (-27.5, -28.415) -> (-27.5, -24.815)
  line L30 (-24.5, -41.415) -> (-20.9, -41.415)
  line L31 (-1.8, -41.415) -> (1.8, -41.415)
  line L32 (20.9, -41.415) -> (24.5, -41.415)
  constraint coincident L20 L28.start
  constraint coincident L0.start L23.end
  constraint coincident L16.end L17.start
  constraint coincident L19.end L20.start
  constraint coincident L14.end L15.start
  constraint coincident L11.end L12.start
  constraint coincident L10.end L11.start
  constraint coincident L7.end L8.start
  constraint coincident L6.end L7.start
  constraint coincident L3.end L4.start
extrude "Extrude7" add sketch "tab_top" along normal up to surface (10.6 mm away) contours L21 L22 L23 L28 | L17 L18 L19 L29 | L4 L5 L6 L32 | L8 L9 L10 L31 | L12 L13 L14 L30 bodies 2
sketch "roof_high" plane through (0, 0, 16) normal (0, 0, 1) x (-1, 0, 0)
  line L0 (27.5, 41.415) -> (27.5, -41.415)
  line L1 (27.5, -41.415) -> (-27.5, -41.415)
  line L2 (-27.5, -41.415) -> (-27.5, 41.415)
  line L3 (-27.5, 41.415) -> (27.5, 41.415)
  line L4 (-30.5, -44.415) -> (30.45, -44.415)
  line L5 (30.45, -44.415) -> (30.45, 44.365)
  line L6 (30.45, 44.365) -> (-30.5, 44.365)
  line L7 (-30.5, 44.365) -> (-30.5, -44.415)
  line L8 (-30.5, -44.415) -> (30.45, -44.415)
  line L9 (30.45, -44.415) -> (30.45, 8.585)
  line L10 (30.45, 8.585) -> (-30.5, 8.585)
  line L11 (-30.5, 8.585) -> (-30.5, -44.415)
  line L12 (-0.025, 8.585) -> (-0.025, 20.585) construction
  line L13 (-0.025, 20.585) -> (4.975, 20.585)
  line L14 (4.975, 20.585) -> (4.975, 8.585)
  line L15 (-0.025, 20.585) -> (-5.025, 20.585)
  line L16 (-5.025, 20.585) -> (-5.025, 8.585)
  line L17 (4.975, 8.585) -> (30.45, 8.585)
  line L18 (30.45, 8.585) -> (30.45, 44.365)
  line L19 (30.45, 44.365) -> (5.075, 44.365)
  line L20 (-5.025, 20.585) -> (5.075, 20.585)
  line L21 (-0.025, 20.585) -> (-7.525, 20.585)
  line L22 (-7.525, 20.585) -> (-7.525, 41.415)
  line L23 (-0.025, 20.585) -> (7.475, 20.585)
  line L24 (7.475, 20.585) -> (7.475, 41.415)
  line L25 (-7.525, 20.585) -> (-27.5, 20.585)
  line L26 (7.475, 20.585) -> (27.5, 20.585)
  line L27 (7.475, 20.585) -> (7.475, 8.585)
  line L28 (-7.525, 20.585) -> (-7.525, 8.585)
  line L29 (7.475, 8.585) -> (7.475, -41.415) construction
  line L30 (-7.525, 8.585) -> (-7.525, -41.415) construction
  line L31 (7.475, -41.415) -> (7.475, -44.415) construction
  line L32 (-7.525, -41.415) -> (7.475, -41.415)
  line L33 (7.475, -41.415) -> (7.475, -44.415)
  line L34 (7.475, -44.415) -> (-7.525, -44.415)
  line L35 (-7.525, -44.415) -> (-7.525, -41.415)
  line L36 (7.475, -41.415) -> (-7.525, -41.415)
  line L37 (-7.525, -41.415) -> (-7.525, -35.315)
  line L38 (-7.525, -35.315) -> (7.475, -35.315)
  line L39 (7.475, -35.315) -> (7.475, -41.415)
  dimension "d101" = 53
  dimension "d104" = 5
  dimension "d105" = 12
  dimension "d108" = 7.5
  dimension "d109" = 12
  dimension "d110" = 12
  dimension "d125" = 6.1
  constraint horizontal L8
  constraint vertical L9
  constraint horizontal L10
  constraint vertical L11
  constraint coincident L5 L9.end
  constraint coincident L4.start L7.end
  constraint midpoint L10 L12.start
  constraint perpendicular L10 L12
  constraint perpendicular L12 L13
  constraint perpendicular L10 L14
  constraint perpendicular L12 L15
  constraint coincident L10 L16.end
  constraint equal L13 L15
  constraint perpendicular L10 L16
  constraint equal L12 L14
  constraint horizontal L17
  constraint vertical L18
  constraint horizontal L19
  constraint coincident L5.end L6.start
  constraint horizontal L20
  constraint perpendicular L16 L21
  constraint coincident L3 L22.end
  constraint perpendicular L3 L22
  constraint perpendicular L12 L23
  constraint equal L21 L23
  constraint coincident L3 L24.end
  constraint perpendicular L3 L24
  constraint coincident L2 L25.end
  constraint perpendicular L2 L25
  constraint coincident L0 L26.end
  constraint perpendicular L0 L26
  constraint perpendicular L10 L27
  constraint perpendicular L25 L28
  constraint coincident L1 L29.end
  constraint perpendicular L1 L29
  constraint coincident L1 L30.end
  constraint perpendicular L1 L30
  constraint perpendicular L8 L31
  constraint horizontal L32
  constraint vertical L33
  constraint horizontal L34
  constraint vertical L35
  constraint horizontal L36
  constraint vertical L37
  constraint horizontal L38
  constraint vertical L39
  constraint coincident L30 L37.end
  measures "d101" distance of L4.end L9.end
  measures "d104" distance of L12.end L13.end
  measures "d105" distance of L13.end L14.end
  measures "d108" distance of L12.end L21.end
  measures "d109" distance of L23.end L27.end
  measures "d110" distance of L21.end L28.end
  measures "d125" distance of L36 L38
extrude "Extrude8" add sketch "roof_high" along normal blind 3 contours L0 L2 L3 L5 L6 L7 L10 L17 L18 L19 | L0 L3 L24 L26 | L0 L10 L17 L26 L27 | L0 L1 L4 L5 L8 L9 L10 L17 L33 | L0 L1 L2 L10 L17 L37 L38 L39 | L2 L3 L22 L25 | L2 L10 L25 L28 | L1 L4 L8 L32 L33 L34 L35 L36 | L1 L32 L36 L37 L38 L39 | L1 L2 L4 L7 L8 L10 L11 L35 bodies 2
ref_plane "WorkPlane2" through (14.35, 0, 15) normal (0, 0, 1) x (1, 0, 0)
sketch "button_slot" plane through (0, 0, 15) normal (0, 0, 1) x (1, 0, 0)
  line L0 (7.525, -41.415) -> (-7.475, -41.415)
  line L1 (-30.45, -44.365) -> (30.5, -44.365)
  line L2 (30.5, -44.365) -> (30.5, 44.415)
  line L3 (30.5, 44.415) -> (-30.45, 44.415)
  line L4 (-30.45, 44.415) -> (-30.45, -44.365)
  line L5 (-7.475, -41.415) -> (-7.475, -44.365)
  line L6 (-7.475, -44.365) -> (7.525, -44.365)
  line L7 (7.525, -44.365) -> (7.525, -41.415)
  line L8 (-7.475, -41.415) -> (7.525, -41.415)
  line L9 (9.025, -42.915) -> (-8.975, -42.915)
  line L10 (-7.475, -41.415) -> (-8.975, -41.415)
  line L11 (7.525, -41.415) -> (9.025, -41.415)
  line L12 (0.025, -20.585) -> (5.025, -20.585)
  line L13 (5.025, -20.585) -> (-5.075, -20.585)
  line L14 (-4.975, -20.585) -> (-4.975, -8.585)
  line L15 (5.025, -20.585) -> (5.025, -8.585)
  line L16 (5.025, -20.585) -> (5.025, -41.415)
  line L17 (-4.975, -8.585) -> (5.025, -8.585)
  line L18 (5.025, -20.585) -> (5.025, -41.415)
  line L19 (-7.475, -41.415) -> (-7.475, -8.585)
  line L20 (-7.475, -8.585) -> (-4.975, -8.585)
  line L21 (7.525, -41.415) -> (7.525, -8.585)
  line L22 (7.525, -8.585) -> (5.025, -8.585)
  line L23 (-4.975, -20.585) -> (-4.975, -41.415)
  dimension "d114" = -1.5
  constraint coincident L0.end L5.start
  constraint coincident L1 L5.end
  constraint perpendicular L1 L5
  constraint coincident L1 L6.end
  constraint coincident L0.start L7.end
  constraint perpendicular L6 L7
  constraint coincident L12.end L13.start
  constraint coincident L0 L16.end
  constraint perpendicular L0 L16
  constraint coincident L14.end L17.start
  constraint coincident L15.end L17.end
  constraint perpendicular L8 L19
  constraint perpendicular L19 L20
  constraint perpendicular L11 L21
  constraint perpendicular L21 L22
  constraint coincident L14.start L23.start
  constraint coincident L8 L23.end
  constraint perpendicular L8 L23
extrude "Extrude9" cut sketch "button_slot" along normal up to surface (4 mm away) contours L0 L5 L7 L8 L9 | L1 L5 L6 L7 L9 bodies 2
ref_plane "WorkPlane3" through (14.35, 0, 10.3) normal (0, 0, 1) x (1, 0, 0)
sketch "roof_wall" plane through (0, 0, 10.3) normal (0, 0, 1) x (1, 0, 0)
  line L0 (-7.475, -44.365) -> (-7.475, -8.585)
  line L1 (-7.475, -8.585) -> (7.525, -8.585)
  line L2 (7.525, -8.585) -> (7.525, -44.365)
  line L3 (-8.975, -44.365) -> (-8.975, -7.085)
  line L4 (-8.975, -7.085) -> (9.025, -7.085)
  line L5 (9.025, -7.085) -> (9.025, -44.365)
  line L6 (-7.475, -44.365) -> (-8.975, -44.365)
  line L7 (9.025, -44.365) -> (7.525, -44.365)
  line L8 (-7.475, -8.585) -> (-8.975, -8.585)
  line L9 (7.525, -8.585) -> (9.025, -8.585)
  dimension "d118" = -1.5
  constraint coincident L0.start L6.start
  constraint perpendicular L3 L6
  constraint coincident L2.end L7.end
  constraint perpendicular L2 L7
  constraint coincident L0.end L1.start
  constraint coincident L3 L8.end
  constraint perpendicular L3 L8
  constraint coincident L1.end L2.start
  constraint coincident L5 L9.end
  constraint perpendicular L5 L9
extrude "Extrude11" add sketch "roof_wall" along normal up to surface (8.7 mm away) contours L0 L3 L6 L8 | L2 L5 L7 L9 bodies 2
extrude "Extrude12" add sketch "button_slot" against normal up to surface (4.7 mm away) contours L0 L8 L15 L16 L18 L21 L22 | L0 L8 L14 L19 L20 L23 bodies 2
sketch "roof_wall2" plane through (0, 0, 16) normal (0, 0, -1) x (1, 0, 0)
  line L0 (9.025, 41.415) -> (9.025, 8.585)
  line L1 (9.025, 8.585) -> (7.525, 8.585)
  line L2 (7.525, 8.585) -> (-7.475, 8.585)
  line L3 (-7.475, 8.585) -> (-8.975, 8.585)
  line L4 (-8.975, 8.585) -> (-8.975, 41.415)
  line L5 (-8.975, 41.415) -> (-27.5, 41.415)
  line L6 (-27.5, 41.415) -> (-27.5, -41.415)
  line L7 (-27.5, -41.415) -> (27.5, -41.415)
  line L8 (27.5, -41.415) -> (27.5, 41.415)
  line L9 (27.5, 41.415) -> (9.025, 41.415)
  line L10 (-8.975, 44.365) -> (-8.975, 7.085)
  line L11 (-8.975, 7.085) -> (9.025, 7.085)
  line L12 (9.025, 7.085) -> (9.025, 44.365)
  line L13 (-7.475, 8.585) -> (-8.975, 8.585)
  line L14 (-7.475, 8.585) -> (7.525, 8.585)
  line L15 (7.525, 8.585) -> (9.025, 8.585)
  line L16 (-8.975, 7.085) -> (9.025, 7.085)
  line L17 (9.025, 7.085) -> (9.025, 8.585)
  line L18 (9.025, 8.585) -> (-8.975, 8.585)
  line L19 (-8.975, 8.585) -> (-8.975, 7.085)
  constraint horizontal L16
  constraint vertical L17
  constraint horizontal L18
  constraint vertical L19
  constraint coincident L0.end L1.start
  constraint coincident L10.end L11.start